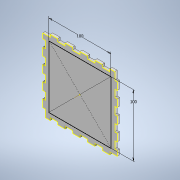
# Autodesk Inventor part: Lukt_hlidarplata
Saved by Autodesk Inventor 2021 (Build 250183000, 183)
## iProperties
Created: 2023-02-22
Part Number: Lukt_hlidarplata
Material: Generic
Document SubType Name: Modeling
Designer: frost
Density: 1 g/cm^3
Appearance: Default
width: 120.000 mm
height: 120.000 mm
thickness: 4.000 mm
finger: 12.000 mm
kerf: 0.220 mm
nr_width: 10.000 ul
nr_height: 10.000 ul
Author: frost
Autodesk Inventor part; units mm, degrees
ref_plane "YZ Plane" through (0, 0, 0) normal (1, 0, 0) x (0, 1, 0)
ref_plane "XZ Plane" through (0, 0, 0) normal (0, 1, 0) x (-1, 0, 0)
ref_plane "XY Plane" through (0, 0, 0) normal (0, 0, 1) x (1, 0, 0)
sketch "Sketch1" plane through (0, 0, 0) normal (0, 0, 1) x (1, 0, 0)
  line L0 (-60, -60) -> (60, -60)
  line L1 (60, -60) -> (60, 60)
  line L2 (60, 60) -> (-60, 60)
  line L3 (-60, 60) -> (-60, -60)
  line L4 (-30, 60) -> (-24.8931, 60)
  point P0 (0, 0)
  dimension "d0" = 120
  dimension "d1" = 120
  dimension "d2" = 60
  dimension "d3" = 60
  constraints: 10 end point, 2 horizontal, 2 parallel, 1 perpendicular, 1 point on line
  measures "d0" distance of L1.end L2.end
  measures "d1" distance of L0.end L1.end
  measures "d2" distance from line of L3 point (0, 0)
  measures "d3" distance from line of L2 point (0, 0)
extrude "Extrusion1" add sketch "Sketch1" along normal mid plane 4
sketch "Sketch3" plane through (-60, 60, 2) normal (0, 1, 0) x (1, 0, 0)
  line L0 (120, 0) -> (0, 0) projected
  line L1 (0, 4) -> (120, 4) projected
  line L2 (0, 0) -> (12, 0)
  line L3 (12, 0) -> (12, 4)
  line L4 (12, 4) -> (0, 4)
  line L5 (0, 4) -> (0, 0)
  line L6 (0, 4) -> (0, 0) projected
  point P0 (60, 2)
  point P1 (12, 0)
  dimension "d17" = 0
  dimension "d18" = 12
  constraints: 8 end point, 2 parallel, 2 point on line, 1 horizontal, 1 perpendicular
  measures "d17" distance between parallel lines of L6 L5
  measures "d18" distance between parallel lines of L3 L5
extrude "Extrusion2" cut sketch "Sketch3" against normal blind 4
pattern_linear "side_top" count 5 spacing 24 along (1, 0, 0) of "Extrusion2"
sketch "Sketch4" plane through (-60, 56, -2) normal (-1, 0, 0) x (0, 0, 1)
  line L0 (4, 0) -> (4, -116) projected
  line L1 (0, -116) -> (4, -116)
  line L2 (4, -116) -> (4, -104)
  line L3 (4, -104) -> (0, -104)
  line L4 (0, -104) -> (0, -116)
  line L5 (0, -116) -> (4, -116) projected
  point P0 (2, -56)
  point P1 (4, -112)
  point P2 (4, -104)
  dimension "d49" = 4
  dimension "d50" = 12
  dimension "d51" = 0
  dimension "d52" = 0
  constraints: 8 end point, 2 parallel, 1 horizontal, 1 perpendicular
  measures "d49" distance of L2.end L3.end
  measures "d50" distance of L3.end L1.start
  measures "d51" distance between parallel lines of L0 L2
  measures "d52" distance between parallel lines of L5 L1
extrude "Extrusion3" cut sketch "Sketch4" against normal blind 4
pattern_circular "side_bottom" count 2 over 360 about axis through (0, 0, -10) along (0, 0, 1) of "Extrusion2", "side_top"
pattern_linear "side_left" count 5 spacing 24 along (0, 1, 0) of "Extrusion3"
pattern_circular "side_right" count 2 over 360 about axis through (0, 0, -10) along (0, 0, 1) of "Extrusion3", "side_left"
sketch "Sketch6" plane through (0, 0, 2) normal (0, 0, 1) x (1, 0, 0)
  line L0 (56, -36) -> (60, -36) projected
  line L1 (60, -36) -> (60, -24) projected
  line L2 (60, -24) -> (56, -24) projected
  line L3 (56, -24) -> (56, -12) projected
  line L4 (56, -12) -> (60, -12) projected
  line L5 (60, -12) -> (60, 0) projected
  line L6 (60, 0) -> (56, 0) projected
  line L7 (56, 0) -> (56, 12) projected
  line L8 (56, 12) -> (60, 12) projected
  line L9 (60, 12) -> (60, 24) projected
  line L10 (60, 24) -> (56, 24) projected
  line L11 (56, 24) -> (56, 36) projected
  line L12 (56, 36) -> (60, 36) projected
  line L13 (60, 36) -> (60, 48) projected
  line L14 (60, 48) -> (56, 48) projected
  line L15 (56, 48) -> (56, 60) projected
  line L16 (56, 60) -> (48, 60) projected
  line L17 (48, 60) -> (48, 56) projected
  line L18 (48, 56) -> (36, 56) projected
  line L19 (36, 56) -> (36, 60) projected
  line L20 (36, 60) -> (24, 60) projected
  line L21 (24, 60) -> (24, 56) projected
  line L22 (24, 56) -> (12, 56) projected
  line L23 (12, 56) -> (12, 60) projected
  line L24 (12, 60) -> (0, 60) projected
  line L25 (0, 60) -> (0, 56) projected
  line L26 (0, 56) -> (-12, 56) projected
  line L27 (-12, 56) -> (-12, 60) projected
  line L28 (-12, 60) -> (-24, 60) projected
  line L29 (-24, 60) -> (-24, 56) projected
  line L30 (-24, 56) -> (-36, 56) projected
  line L31 (-36, 56) -> (-36, 60) projected
  line L32 (-36, 60) -> (-48, 60) projected
  line L33 (-48, 60) -> (-48, 56) projected
  line L34 (-48, 56) -> (-60, 56) projected
  line L35 (-60, 56) -> (-60, 48) projected
  line L36 (-60, 48) -> (-56, 48) projected
  line L37 (-56, 48) -> (-56, 36) projected
  line L38 (-56, 36) -> (-60, 36) projected
  line L39 (-60, 36) -> (-60, 24) projected
  line L40 (-60, 24) -> (-56, 24) projected
  line L41 (-56, 24) -> (-56, 12) projected
  line L42 (-56, 12) -> (-60, 12) projected
  line L43 (-60, 12) -> (-60, 0) projected
  line L44 (-60, 0) -> (-56, 0) projected
  line L45 (-56, 0) -> (-56, -12) projected
  line L46 (-56, -12) -> (-60, -12) projected
  line L47 (-60, -12) -> (-60, -24) projected
  line L48 (-60, -24) -> (-56, -24) projected
  line L49 (-56, -24) -> (-56, -36) projected
  line L50 (-56, -36) -> (-60, -36) projected
  line L51 (-60, -36) -> (-60, -48) projected
  line L52 (-60, -48) -> (-56, -48) projected
  line L53 (-56, -48) -> (-56, -60) projected
  line L54 (-56, -60) -> (-48, -60) projected
  line L55 (-48, -60) -> (-48, -56) projected
  line L56 (-48, -56) -> (-36, -56) projected
  line L57 (-36, -56) -> (-36, -60) projected
  line L58 (-36, -60) -> (-24, -60) projected
  line L59 (-24, -60) -> (-24, -56) projected
  line L60 (-24, -56) -> (-12, -56) projected
  line L61 (-12, -56) -> (-12, -60) projected
  line L62 (-12, -60) -> (0, -60) projected
  line L63 (0, -60) -> (0, -56) projected
  line L64 (0, -56) -> (12, -56) projected
  line L65 (12, -56) -> (12, -60) projected
  line L66 (12, -60) -> (24, -60) projected
  line L67 (24, -60) -> (24, -56) projected
  line L68 (24, -56) -> (36, -56) projected
  line L69 (36, -56) -> (36, -60) projected
  line L70 (36, -60) -> (48, -60) projected
  line L71 (48, -60) -> (48, -56) projected
  line L72 (48, -56) -> (60, -56) projected
  line L73 (60, -56) -> (60, -48) projected
  line L74 (60, -48) -> (56, -48) projected
  line L75 (56, -48) -> (56, -36) projected
  line L76 (-48.11, 60.11) -> (-35.89, 60.11)
  line L77 (-35.89, 60.11) -> (-35.89, 56.11)
  line L78 (-35.89, 56.11) -> (-24.11, 56.11)
  line L79 (-24.11, 56.11) -> (-24.11, 60.11)
  line L80 (-24.11, 60.11) -> (-11.89, 60.11)
  line L81 (-11.89, 60.11) -> (-11.89, 56.11)
  line L82 (-11.89, 56.11) -> (-0.11, 56.11)
  line L83 (-0.11, 56.11) -> (-0.11, 60.11)
  line L84 (-0.11, 60.11) -> (12.11, 60.11)
  line L85 (12.11, 60.11) -> (12.11, 56.11)
  line L86 (12.11, 56.11) -> (23.89, 56.11)
  line L87 (23.89, 56.11) -> (23.89, 60.11)
  line L88 (23.89, 60.11) -> (36.11, 60.11)
  line L89 (36.11, 60.11) -> (36.11, 56.11)
  line L90 (36.11, 56.11) -> (47.89, 56.11)
  line L91 (47.89, 56.11) -> (47.89, 60.11)
  line L92 (47.89, 60.11) -> (56.11, 60.11)
  line L93 (56.11, 60.11) -> (56.11, 48.11)
  line L94 (56.11, 48.11) -> (60.11, 48.11)
  line L95 (60.11, 48.11) -> (60.11, 35.89)
  line L96 (60.11, 35.89) -> (56.11, 35.89)
  line L97 (56.11, 35.89) -> (56.11, 24.11)
  line L98 (56.11, 24.11) -> (60.11, 24.11)
  line L99 (60.11, 24.11) -> (60.11, 11.89)
  line L100 (60.11, 11.89) -> (56.11, 11.89)
  line L101 (56.11, 11.89) -> (56.11, 0.11)
  line L102 (56.11, 0.11) -> (60.11, 0.11)
  line L103 (60.11, 0.11) -> (60.11, -12.11)
  line L104 (60.11, -12.11) -> (56.11, -12.11)
  line L105 (56.11, -12.11) -> (56.11, -23.89)
  line L106 (56.11, -23.89) -> (60.11, -23.89)
  line L107 (60.11, -23.89) -> (60.11, -36.11)
  line L108 (60.11, -36.11) -> (56.11, -36.11)
  line L109 (56.11, -36.11) -> (56.11, -47.89)
  line L110 (56.11, -47.89) -> (60.11, -47.89)
  line L111 (60.11, -47.89) -> (60.11, -56.11)
  line L112 (60.11, -56.11) -> (48.11, -56.11)
  line L113 (48.11, -56.11) -> (48.11, -60.11)
  line L114 (48.11, -60.11) -> (35.89, -60.11)
  line L115 (35.89, -60.11) -> (35.89, -56.11)
  line L116 (35.89, -56.11) -> (24.11, -56.11)
  line L117 (24.11, -56.11) -> (24.11, -60.11)
  line L118 (24.11, -60.11) -> (11.89, -60.11)
  line L119 (11.89, -60.11) -> (11.89, -56.11)
  line L120 (11.89, -56.11) -> (0.11, -56.11)
  line L121 (0.11, -56.11) -> (0.11, -60.11)
  line L122 (0.11, -60.11) -> (-12.11, -60.11)
  line L123 (-12.11, -60.11) -> (-12.11, -56.11)
  line L124 (-12.11, -56.11) -> (-23.89, -56.11)
  line L125 (-23.89, -56.11) -> (-23.89, -60.11)
  line L126 (-23.89, -60.11) -> (-36.11, -60.11)
  line L127 (-36.11, -60.11) -> (-36.11, -56.11)
  line L128 (-36.11, -56.11) -> (-47.89, -56.11)
  line L129 (-47.89, -56.11) -> (-47.89, -60.11)
  line L130 (-47.89, -60.11) -> (-56.11, -60.11)
  line L131 (-56.11, -60.11) -> (-56.11, -48.11)
  line L132 (-56.11, -48.11) -> (-60.11, -48.11)
  line L133 (-60.11, -48.11) -> (-60.11, -35.89)
  line L134 (-60.11, -35.89) -> (-56.11, -35.89)
  line L135 (-56.11, -35.89) -> (-56.11, -24.11)
  line L136 (-56.11, -24.11) -> (-60.11, -24.11)
  line L137 (-60.11, -24.11) -> (-60.11, -11.89)
  line L138 (-60.11, -11.89) -> (-56.11, -11.89)
  line L139 (-56.11, -11.89) -> (-56.11, -0.11)
  line L140 (-56.11, -0.11) -> (-60.11, -0.11)
  line L141 (-60.11, -0.11) -> (-60.11, 12.11)
  line L142 (-60.11, 12.11) -> (-56.11, 12.11)
  line L143 (-56.11, 12.11) -> (-56.11, 23.89)
  line L144 (-56.11, 23.89) -> (-60.11, 23.89)
  line L145 (-60.11, 23.89) -> (-60.11, 36.11)
  line L146 (-60.11, 36.11) -> (-56.11, 36.11)
  line L147 (-56.11, 36.11) -> (-56.11, 47.89)
  line L148 (-56.11, 47.89) -> (-60.11, 47.89)
  line L149 (-60.11, 47.89) -> (-60.11, 56.11)
  line L150 (-60.11, 56.11) -> (-48.11, 56.11)
  line L151 (-48.11, 56.11) -> (-48.11, 60.11)
  point P0 (0, 0)
  dimension "d59" = 0.11
  constraints: 152 end point, 75 other
  measures "d59" distance between parallel lines of L32 L76
extrude "Extrusion5" add sketch "Sketch6" against normal blind 4 contours L75 L74 L73 L72 L71 L70 L69 L68 L67 L66 L65 L64 L63 L62 L61 L60 L59 L58 L57 L56 L55 L54 L53 L52 L51 L50 L49 L48 L47 L46 L45 L44 L43 L42 L41 L40 L39 L38 L37 L36 L35 L34 L33 L32 L31 L30 L29 L28 L27 L26 L25 L24 L23 L22 L21 L20 L19 L18 L17 L16 L15 L14 L13 L12 L11 L10 L9 L8 L7 L6 L5 L4 L3 L2 L1 L0 | L76 L77 L78 L79 L80 L81 L82 L83 L84 L85 L86 L87 L88 L89 L90 L91 L92 L93 L94 L95 L96 L97 L98 L99 L100 L101 L102 L103 L104 L105 L106 L107 L108 L109 L110 L111 L112 L113 L114 L115 L116 L117 L118 L119 L120 L121 L122 L123 L124 L125 L126 L127 L128 L129 L130 L131 L132 L133 L134 L135 L136 L137 L138 L139 L140 L141 L142 L143 L144 L145 L146 L147 L148 L149 L150 L151
sketch "Sketch7" plane through (0, 0, 2) normal (0, 0, 1) x (1, 0, 0)
  line L0 (-48.11, 56.11) -> (-60.11, 56.11) projected
  line L1 (-60.11, 56.11) -> (-60.11, 47.89) projected
  line L2 (-60.11, 47.89) -> (-56.11, 47.89) projected
  line L3 (-56.11, 47.89) -> (-56.11, 36.11) projected
  line L4 (-56.11, 36.11) -> (-60.11, 36.11) projected
  line L5 (-60.11, 36.11) -> (-60.11, 23.89) projected
  line L6 (-60.11, 23.89) -> (-56.11, 23.89) projected
  line L7 (-56.11, 23.89) -> (-56.11, 12.11) projected
  line L8 (-56.11, 12.11) -> (-60.11, 12.11) projected
  line L9 (-60.11, 12.11) -> (-60.11, -0.11) projected
  line L10 (-60.11, -0.11) -> (-56.11, -0.11) projected
  line L11 (-56.11, -0.11) -> (-56.11, -11.89) projected
  line L12 (-56.11, -11.89) -> (-60.11, -11.89) projected
  line L13 (-60.11, -11.89) -> (-60.11, -24.11) projected
  line L14 (-60.11, -24.11) -> (-56.11, -24.11) projected
  line L15 (-56.11, -24.11) -> (-56.11, -35.89) projected
  line L16 (-56.11, -35.89) -> (-60.11, -35.89) projected
  line L17 (-60.11, -35.89) -> (-60.11, -48.11) projected
  line L18 (-60.11, -48.11) -> (-56.11, -48.11) projected
  line L19 (-56.11, -48.11) -> (-56.11, -60.11) projected
  line L20 (-56.11, -60.11) -> (-47.89, -60.11) projected
  line L21 (-47.89, -60.11) -> (-47.89, -56.11) projected
  line L22 (-47.89, -56.11) -> (-36.11, -56.11) projected
  line L23 (-36.11, -56.11) -> (-36.11, -60.11) projected
  line L24 (-36.11, -60.11) -> (-23.89, -60.11) projected
  line L25 (-23.89, -60.11) -> (-23.89, -56.11) projected
  line L26 (-23.89, -56.11) -> (-12.11, -56.11) projected
  line L27 (-12.11, -56.11) -> (-12.11, -60.11) projected
  line L28 (-12.11, -60.11) -> (0.11, -60.11) projected
  line L29 (0.11, -60.11) -> (0.11, -56.11) projected
  line L30 (0.11, -56.11) -> (11.89, -56.11) projected
  line L31 (11.89, -56.11) -> (11.89, -60.11) projected
  line L32 (11.89, -60.11) -> (24.11, -60.11) projected
  line L33 (24.11, -60.11) -> (24.11, -56.11) projected
  line L34 (24.11, -56.11) -> (35.89, -56.11) projected
  line L35 (35.89, -56.11) -> (35.89, -60.11) projected
  line L36 (35.89, -60.11) -> (48.11, -60.11) projected
  line L37 (48.11, -60.11) -> (48.11, -56.11) projected
  line L38 (48.11, -56.11) -> (60.11, -56.11) projected
  line L39 (60.11, -56.11) -> (60.11, -47.89) projected
  line L40 (60.11, -47.89) -> (56.11, -47.89) projected
  line L41 (56.11, -47.89) -> (56.11, -36.11) projected
  line L42 (56.11, -36.11) -> (60.11, -36.11) projected
  line L43 (60.11, -36.11) -> (60.11, -23.89) projected
  line L44 (60.11, -23.89) -> (56.11, -23.89) projected
  line L45 (56.11, -23.89) -> (56.11, -12.11) projected
  line L46 (56.11, -12.11) -> (60.11, -12.11) projected
  line L47 (60.11, -12.11) -> (60.11, 0.11) projected
  line L48 (60.11, 0.11) -> (56.11, 0.11) projected
  line L49 (56.11, 0.11) -> (56.11, 11.89) projected
  line L50 (56.11, 11.89) -> (60.11, 11.89) projected
  line L51 (60.11, 11.89) -> (60.11, 24.11) projected
  line L52 (60.11, 24.11) -> (56.11, 24.11) projected
  line L53 (56.11, 24.11) -> (56.11, 35.89) projected
  line L54 (56.11, 35.89) -> (60.11, 35.89) projected
  line L55 (60.11, 35.89) -> (60.11, 48.11) projected
  line L56 (60.11, 48.11) -> (56.11, 48.11) projected
  line L57 (56.11, 48.11) -> (56.11, 60.11) projected
  line L58 (56.11, 60.11) -> (47.89, 60.11) projected
  line L59 (47.89, 60.11) -> (47.89, 56.11) projected
  line L60 (47.89, 56.11) -> (36.11, 56.11) projected
  line L61 (36.11, 56.11) -> (36.11, 60.11) projected
  line L62 (36.11, 60.11) -> (23.89, 60.11) projected
  line L63 (23.89, 60.11) -> (23.89, 56.11) projected
  line L64 (23.89, 56.11) -> (12.11, 56.11) projected
  line L65 (12.11, 56.11) -> (12.11, 60.11) projected
  line L66 (12.11, 60.11) -> (-0.11, 60.11) projected
  line L67 (-0.11, 60.11) -> (-0.11, 56.11) projected
  line L68 (-0.11, 56.11) -> (-11.89, 56.11) projected
  line L69 (-11.89, 56.11) -> (-11.89, 60.11) projected
  line L70 (-11.89, 60.11) -> (-24.11, 60.11) projected
  line L71 (-24.11, 60.11) -> (-24.11, 56.11) projected
  line L72 (-24.11, 56.11) -> (-35.89, 56.11) projected
  line L73 (-35.89, 56.11) -> (-35.89, 60.11) projected
  line L74 (-35.89, 60.11) -> (-48.11, 60.11) projected
  line L75 (-48.11, 60.11) -> (-48.11, 56.11) projected
  line L76 (-50, -50) -> (50, -50)
  line L77 (50, -50) -> (50, 50)
  line L78 (50, 50) -> (-50, 50)
  line L79 (-50, 50) -> (-50, -50)
  line L80 (-50, -50) -> (50, 50) construction
  line L81 (50, -50) -> (-50, 50) construction
  point P0 (0, 0)
  dimension "d62" = 100
  dimension "d63" = 100
  constraints: 12 end point, 2 midpoint, 2 parallel, 1 horizontal, 1 perpendicular
  measures "d62" distance of L77.end L78.end
  measures "d63" distance of L76.end L77.end
equation "\"d0\" = width"
equation "\"d1\" = height"
equation "\"d2\" = 0.5 * width"
equation "\"d3\" = 0.5 * height"
equation "\"d4\" = thickness"
equation "\"d18\" = finger"
equation "\"d19\" = thickness"
equation "\"d23\" = 2 * finger"
equation "\"d49\" = thickness"
equation "\"d50\" = finger"
equation "\"d28\" = thickness"
equation "\"d55\" = 2 * finger"
equation "\"d59\" = 0.5 * kerf"
equation "\"d60\" = thickness"
equation "\"width\" = 120"
equation "\"height\" = 120"
equation "\"thickness\" = 4"
equation "\"finger\" = 3 * thickness"
equation "\"kerf\" = 0.22"
body "Solid1"
